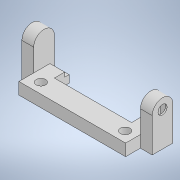
# Autodesk Inventor part: Крепление OpenMV
Saved by Autodesk Inventor 2020 (Build 240168000, 168)
## iProperties
Created: 2021-07-06
Part Number: Крепление OpenMV
Material: Типовые
Document SubType Name: Modeling
Designer: Антон
Density: 1 g/cm^3
Appearance: По умолчанию
Author: Антон
Autodesk Inventor part; units mm, degrees
ref_plane "YZ Plane" through (0, 0, 0) normal (1, 0, 0) x (0, 1, 0)
ref_plane "XZ Plane" through (0, 0, 0) normal (0, 1, 0) x (-1, 0, 0)
ref_plane "XY Plane" through (0, 0, 0) normal (0, 0, 1) x (1, 0, 0)
sketch "Эскиз1" plane through (0, 0, 0) normal (0, 1, 0) x (-1, 0, 0)
  line L0 (0, 0) -> (36.1, 0)
  line L1 (36.1, 0) -> (36.1, -7)
  line L2 (36.1, -7) -> (0, -7)
  line L3 (0, -7) -> (0, 0)
  line L4 (36.1, -7) -> (31.1, -7)
  line L5 (31.1, -7) -> (31.1, -12)
  line L6 (31.1, -12) -> (36.1, -12)
  line L7 (36.1, -12) -> (36.1, -7)
  line L8 (36.1, -12) -> (40.1, -12)
  line L9 (40.1, -12) -> (40.1, -5)
  line L10 (40.1, -5) -> (36.1, -5)
  line L11 (36.1, -5) -> (36.1, -12)
  line L12 (18.05, 0) -> (18.05, -7) construction
  line L13 (0, -7) -> (5, -7)
  line L14 (5, -7) -> (5, -12)
  line L15 (5, -12) -> (0, -12)
  line L16 (0, -12) -> (0, -7)
  line L17 (0, -12) -> (-4, -12)
  line L18 (-4, -12) -> (-4, -5)
  line L19 (-4, -5) -> (0, -5)
  line L20 (0, -5) -> (0, -12)
  point P0 (31.1, -7)
  point P1 (0, -5)
  point P2 (36.1, -5)
  dimension "d0" = 36.1
  dimension "d1" = 7
  dimension "d12" = 5
  dimension "d13" = 5
  dimension "d14" = 4
  dimension "d15" = 7
  constraints: 42 end point, 6 parallel, 6 symmetric about line, 3 horizontal, 3 perpendicular, 2 midpoint
  measures "d0" distance of L1.end L2.end
  measures "d1" distance of L0.end L1.end
  measures "d12" distance of L5.end L6.end
  measures "d13" distance of L4.end L5.end
  measures "d14" distance of L10.end L9.end
  measures "d15" distance of L9.end L8.end
extrude "Выдавливание1" add sketch "Эскиз1" along normal blind 4
sketch "Эскиз2" plane through (0, 0, 0) normal (0, -1, 0) x (1, 0, 0)
  line L0 (-36.1, 0) -> (0, 0) construction
  line L1 (-17.75, 0) -> (-18.05, -7) construction
  line L2 (-5, -7) -> (-31.1, -7) construction
  line L3 (-32.15, -3.5) -> (-3.65, -3.5) construction
  point P0 (-35.5, 0)
  point P1 (0, -7)
  point P2 (-35.5, -7)
  point P3 (-17.9, -3.5)
  dimension "d4" = 28.5
  constraints: 4 end point, 3 midpoint, 1 horizontal, 1 point on line
  measures "d4" distance of L3.start L3.end
hole "Отверстие1" at (-32.15, 0, -3.5) at (-3.65, 0, -3.5) direction (0, 1, 0) diameter 3.2 end through all countersink diameter 6 countersink angle 90
sketch "Эскиз3" plane through (0, 4, 0) normal (0, 1, 0) x (1, 0, 0)
  line L0 (-40.1, 5) -> (-36.1, 5) projected
  line L1 (-36.1, 5) -> (-36.1, 12)
  line L2 (-31.1, 12) -> (-40.1, 12) projected
  line L3 (0, 5) -> (4, 5) projected
  line L4 (0, 5) -> (0, 12)
  line L5 (4, 12) -> (-5, 12) projected
  line L6 (4, 5) -> (4, 12) projected
  line L7 (-40.1, 12) -> (-40.1, 5) projected
  point P0 (0, 0)
  constraints: 4 end point, 2 point on line, 2 vertical
extrude "Выдавливание2" add sketch "Эскиз3" along normal blind 11.05
fillet "Сопряжение1" radius 3.5 4 edges at (-38.1, 15.05, -5) (-38.1, 15.05, -12) (2, 15.05, -5) (2, 15.05, -12)
sketch "Эскиз5" plane through (-40.1, 0, -12) normal (-1, 0, 0) x (0, 0, 1)
  arc A0 (7, 11.55) -> (0, 11.55) centre (3.5, 11.55) ccw projected
  arc A1 (7, 11.55) -> (0, 11.55) centre (3.5, 11.55) ccw projected
  point P0 (12, 0)
hole "Отверстие2" at (-40.1, 11.55, -8.5) direction (1, 0, 0) diameter 3.1 depth 3.5
sketch "Эскиз6" plane through (4, 0, -5) normal (1, 0, 0) x (0, 0, -1)
  arc A0 (7, 11.55) -> (0, 11.55) centre (3.5, 11.55) ccw projected
  point P0 (-5, 0)
hole "Отверстие3" at (4, 11.55, -8.5) direction (-1, 0, 0) diameter 3.1 depth 3.5
sketch "Эскиз7" plane through (-40.1, 0, -12) normal (-1, 0, 0) x (0, 0, 1)
  circle A0 centre (3.5, 11.55) radius 1.55 projected
  line L0 (0.7, 13.1666) -> (3.5, 14.7832)
  line L1 (3.5, 14.7832) -> (6.3, 13.1666)
  line L2 (6.3, 13.1666) -> (6.3, 9.9334)
  line L3 (6.3, 9.9334) -> (3.5, 8.3168)
  line L4 (3.5, 8.3168) -> (0.7, 9.9334)
  line L5 (0.7, 9.9334) -> (0.7, 13.1666)
  line L6 (0, 0) -> (0, 11.55) projected
  line L7 (0.7, 9.9334) -> (6.3, 9.9334)
  line L8 (6.3, 9.9334) -> (6.3, 0)
  line L9 (6.3, 0) -> (0.7, 0)
  line L10 (0.7, 0) -> (0.7, 9.9334)
  line L11 (0, 0) -> (7, 0) projected
  point P0 (12, 0)
  point P1 (3.5, 11.55)
  dimension "d33" = 5.6
  constraints: 20 end point, 3 parallel, 2 collinear, 1 coincident, 1 horizontal, 1 perpendicular, 13 other
  measures "d33" distance between parallel lines of L5 L2
extrude "Выдавливание3" cut sketch "Эскиз7" along normal blind 3 from surface at -3.5 contours A0 | L0 L1 L2 L7 L5 | L7 L3 L4 | L4 L3 L8 L9 L10
extrude "Выдавливание4" cut sketch "Эскиз7" against normal blind 3 from surface at -40.6 contours A0 | L0 L1 L2 L7 L5 | L7 L3 L4 | L4 L3 L8 L9 L10
sketch "Эскиз8" plane through (0, 4, 0) normal (0, 1, 0) x (1, 0, 0)
  line L0 (-31.1, 7) -> (-31.1, 12) projected
  line L1 (-31.1, 12) -> (-36.1, 12)
  line L2 (-36.1, 12) -> (-36.1, 10.5)
  line L3 (-36.1, 10.5) -> (-31.1, 10.5)
  line L4 (-31.1, 10.5) -> (-31.1, 12)
  line L5 (-36.1, 12) -> (-36.1, 5) projected
  point P0 (0, 0)
  dimension "d38" = 1.5
  constraints: 8 end point, 2 parallel, 1 collinear, 1 horizontal, 1 perpendicular
  measures "d38" distance of L2.end L1.end
extrude "Выдавливание5" cut sketch "Эскиз8" against normal blind 1.5
